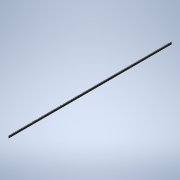
# Autodesk Inventor part: 20_Belt_450mm
Saved by Autodesk Inventor 2022.2 (Build 262287010, 287A)
## iProperties
Created: 2022-04-30
Part Number: 20_Belt_450mm
Material: Generisch
Document SubType Name: Modeling
Designer: MXBD
Density: 1 g/cm^3
Appearance: Schwarz
Author: MXBD
Autodesk Inventor part; units mm, degrees
ref_plane "YZ Plane" through (0, 0, 0) normal (1, 0, 0) x (0, 1, 0)
ref_plane "XZ Plane" through (0, 0, 0) normal (0, 1, 0) x (-1, 0, 0)
ref_plane "XY Plane" through (0, 0, 0) normal (0, 0, 1) x (1, 0, 0)
sketch "Skizze1" plane through (0, 0, 0) normal (0, 1, 0) x (-1, 0, 0)
  line L0 (-0.75, -225) -> (0.75, -225)
  line L1 (0.75, -225) -> (0.75, 225)
  line L2 (0.75, 225) -> (-0.75, 225)
  line L3 (-0.75, 225) -> (-0.75, -225)
  line L4 (-0.75, -225) -> (0.75, 225) construction
  line L5 (0.75, -225) -> (-0.75, 225) construction
  point P0 (0, 0)
  dimension "d0" = 1.5
  dimension "d1" = 450
  constraints: 12 end point, 2 midpoint, 2 parallel, 1 horizontal, 1 perpendicular
  measures "d0" distance of L2.end L1.end
  measures "d1" distance of L1.end L0.end
extrude "Extrusion1" add sketch "Skizze1" along normal blind 6
